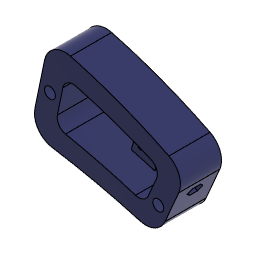
Tibia support middle v12 (Autodesk Fusion 360 design; units mm, degrees)
Autodesk Fusion 360 part; units mm, degrees
sketch "Sketch1" plane through (0, 0, 0) normal (0, 1, 0) x (1, 0, 0)
  line L0 (159.1401, 45.7067) -> (169.6952, 30.6325) construction
  line L1 (-17.5, 10) -> (-10.1, 10)
  line L2 (-18.6, 18.5) -> (-18.6, -18.5)
  line L3 (-17.5, 10) -> (-18.6, 10)
  circle A0 centre (0, 0) radius 2.5
  line L4 (74.5974, 20.8368) -> (81.7385, -13.7478)
  arc A1 (38.4, 18.5) -> (169.9824, 51.1436) centre (38.4, 300.018) ccw
  line L5 (169.9824, 51.1436) -> (178.5861, 38.8564)
  arc A2 (37.3, 10) -> (161.7212, 42.0206) centre (37.3, 267.7398) ccw
  line L6 (-10.1, -10) -> (29.9, -10)
  line L7 (-10.1, 10) -> (-10.1, -10)
  line L8 (29.9, 10) -> (-10.1, 10)
  line L9 (-17.5, -10) -> (-18.6, -10)
  line L10 (-17.5, -10) -> (-17.5, 10)
  line L11 (29.9, -10) -> (29.9, 10)
  line L12 (38.4, -18.5) -> (38.4, 18.5) construction
  line L13 (161.7212, 42.0206) -> (167.1141, 34.3187)
  line L14 (82.53, 21.9804) -> (89.5169, -11.8572)
  line L15 (9.9, -10) -> (9.9, -18.5) construction
  arc A3 (38.4, -18.5) -> (178.5861, 38.8564) centre (38.4, 181.4943) ccw
  line L16 (124.5058, 8.7395) -> (125.8994, 25.7068) construction
  line L17 (0, 0) -> (174.2843, 45) construction
  line L18 (-18.6, -18.5) -> (38.4, -18.5)
  line L19 (115.6359, 29.3023) -> (127.2705, 2.3303)
  line L20 (-10.1, -10) -> (-17.5, -10)
  line L21 (-10.1, 10) -> (-10.1, -10)
  line L22 (169.6952, 30.6325) -> (169.9824, 51.1436) construction
  line L23 (29.9, 10) -> (29.9, -10)
  line L24 (123.3477, 31.6223) -> (134.3836, 6.0382)
  arc A4 (37.3, -10) -> (167.1141, 34.3187) centre (37.3, 202.279) ccw
  line L25 (29.9, -10) -> (37.3, -10)
  line L26 (9.9, 10) -> (9.9, 18.5) construction
  line L27 (159.1401, 45.7067) -> (178.5861, 38.8564) construction
  line L28 (37.3, -10) -> (37.3, 10)
  line L29 (80.0659, -5.6475) -> (84.1183, 14.2879) construction
  line L30 (37.3, 10) -> (29.9, 10)
  line L31 (38.4, 18.5) -> (-18.6, 18.5)
  circle A5 centre (82.0921, 4.3202) radius 2.1
  circle A6 centre (125.2026, 17.2232) radius 2.1
  circle A7 centre (123.6183, 20.8961) radius 2.1
  point P0 (125.2026, 17.2232)
  point P1 (174.2843, 45)
  point P2 (37.3, 0)
  point P3 (82.0921, 4.3202)
  point P4 (-6.8918, -8.1801)
  point P5 (169.8534, 41.9327)
  point P6 (9.9, 13.85)
  dimension "d1" = 5
  dimension "d2" = 10.1
  dimension "d3" = 40
  dimension "d4" = 20
  dimension "d5" = 10
  dimension "d6" = 7.4
  dimension "d7" = 8.5
  dimension "d8" = 8.5
  dimension "d9" = 8.5
  dimension "d10" = 8.5
  dimension "d11" = 180
  dimension "d12" = 45
  dimension "d13" = 35
  dimension "d14" = 15
  dimension "d15" = 12
  dimension "d16" = 4.5
  dimension "d17" = 4.5
  dimension "d18" = 8
  dimension "d19" = 8
  dimension "d20" = 45
  dimension "d21" = 45
  dimension "d22" = 11.667
  dimension "d23" = 11.667
  dimension "d24" = 27.7
  dimension "d25" = 13.85
  dimension "d32" = 4.2
  dimension "d53" = 4
  dimension "d54" = 4
  constraint coincident A0.centre L17.start
  constraint horizontal L6
  constraint vertical L11
  constraint horizontal L8
  constraint vertical L21
  constraint horizontal L20
  constraint vertical L10
  constraint horizontal L1
  constraint vertical L7
  constraint horizontal L25
  constraint vertical L28
  constraint horizontal L30
  constraint vertical L23
  constraint coincident L1.end L7.start
  constraint coincident L8.start L11.end
  constraint equal L20 L25
  constraint horizontal L18
  constraint vertical L12
  constraint horizontal L31
  constraint vertical L2
  constraint coincident P1 L5
  constraint tangent A3 L18
  constraint tangent A1 L31
  constraint midpoint P1 L5
  constraint coincident P1 L17.end
  constraint parallel L0 L5
  constraint coincident L13.end L0
  constraint tangent A4 L25
  constraint coincident A2.end L0
  constraint tangent A2 L30
  constraint coincident L0.end A3
  constraint coincident L0.start A1
  constraint coincident L29.start A4
  constraint coincident L29.end A2
  constraint parallel L4 L14
  constraint coincident L16.start A4
  constraint coincident L16.end A2
  constraint parallel L19 L24
  constraint midpoint P3 L29
  constraint midpoint P0 L16
  constraint midpoint P2 L28
  constraint coincident L9.end L2
  constraint perpendicular L2 L9
  constraint coincident L3.end L2
  constraint perpendicular L2 L3
  constraint midpoint L15.start L6
  constraint midpoint L15.end L18
  constraint midpoint L26.start L8
  constraint midpoint L26.end L31
  constraint coincident P5 L27
  constraint coincident P5 L22
  constraint coincident P6 L26
  constraint coincident L29.start L4
  constraint coincident L29.end L14
  constraint coincident A3 L19.end
  constraint coincident L16.start L19
  constraint coincident A1 L19.start
  constraint coincident A1 L24.start
  constraint coincident L16.end L24
  constraint coincident A3 L4.end
  constraint coincident A3 L14.end
  constraint coincident A1 L4.start
  constraint coincident A1 L14.start
  constraint coincident A3 L24.end
  constraint coincident P3 A5.centre
  constraint coincident P0 A6.centre
  constraint equal A5 A6
  constraint equal A5 A7
  measures "d1" diameter of A0
  measures "d2" distance of A0.centre L21
  measures "d3" distance of L6.start L6.end
  measures "d4" distance of L8.start L6.end
  measures "d5" distance of A0.centre L6
  measures "d6" distance of L6.start L9.start
  measures "d7" distance of L2 L7
  measures "d8" distance of L11 L12
  measures "d9" distance of L8 L31
  measures "d10" distance of L6 L18
  measures "d11" distance of A0.centre P1
  measures "d12" vertical distance of P1 A0.centre
  measures "d13" angle of L2 L5
  measures "d14" distance of L5.end A1.end
  measures "d15" distance of L0 L5
  measures "d16" distance of L0.end L13.end
  measures "d17" distance of A2.end L0.start
  measures "d18" distance of L4 L14
  measures "d19" distance of L19 L24
  measures "d20" distance of P2 P3
  measures "d21" distance of P0 P3
  measures "d22" angle of L4 L28
  measures "d23" angle of L14 L19
  measures "d24" distance of P4 P6
  measures "d25" vertical distance of A0.centre P6
  measures "d32" diameter of A5
  measures "d53" distance of L24 A7.centre
  measures "d54" distance of P0 A7.centre
  measures "d57" angle of P2
extrude "Extrude1" add sketch "Sketch1" along normal blind 15.75 contours L4 A2 L14 A4 | L4 A1 A2 L14 | L4 L14 A3 A4 | A1 A2 L14 L19 | L14 A3 L19 A4 | A1 A2 L19 L24 | A2 L19 L24 A4 | A3 L19 L24 A4 | A6 A7 picked at (125.6121, 16.5727)
fillet "Fillet1" radius 4 4 edges at (84.1183, 7.875, -14.2879) (87.8714, 7.875, 3.8882) (124.5058, 7.875, -8.7395) (118.3255, 7.875, -23.0672)
fillet "Fillet2" radius 8 4 edges at (81.7385, 7.875, 13.7478) (74.5974, 7.875, -20.8368) (123.3477, 7.875, -31.6223) (134.3836, 7.875, -6.0382)
sketch "Sketch3" plane through (0, 15.75, 0) normal (0, 1, 0) x (-1, 0, 0)
  arc A0 (-127.668, -2.528) -> (-131.4429, -12.8555) centre (-124.0972, -9.6868) ccw
  line L0 (-131.4429, -12.8555) -> (-126.1762, -25.0651)
  arc A1 (-126.1762, -25.0651) -> (-116.608, -29.5815) centre (-118.8305, -21.8964) ccw
  arc A2 (-82.8853, -22.037) -> (-116.608, -29.5815) centre (-38.4, -300.018) ccw
  arc A3 (-82.8853, -22.037) -> (-76.3147, -12.5198) centre (-84.1494, -14.1375) ccw
  line L1 (-76.3147, -12.5198) -> (-80.0619, 5.6279)
  arc A4 (-80.0619, 5.6279) -> (-89.959, 11.7397) centre (-87.8966, 4.0101) ccw
  arc A5 (-89.959, 11.7397) -> (-127.668, -2.528) centre (-38.4, -181.4943) ccw
  circle A6 centre (-82.0921, -4.3202) radius 2.1
  arc A7 (-88.0674, -15.0493) -> (-114.8897, -21.9561) centre (-37.3, -267.7398) ccw
  arc A8 (-119.7668, -19.726) -> (-114.8897, -21.9561) centre (-116.0939, -18.1416) ccw
  line L2 (-119.7668, -19.726) -> (-122.9321, -12.3879)
  arc A9 (-120.8332, -7.1263) -> (-122.9321, -12.3879) centre (-119.2592, -10.8036) ccw
  arc A10 (-91.9713, 2.8391) -> (-120.8332, -7.1263) centre (-37.3, -202.279) ccw
  arc A11 (-87.0237, -0.2171) -> (-91.9713, 2.8391) centre (-90.9411, -1.026) ccw
  line L3 (-87.0237, -0.2171) -> (-84.9379, -10.3188)
  arc A12 (-88.0674, -15.0493) -> (-84.9379, -10.3188) centre (-88.8553, -11.1277) ccw
  line L4 (-114.8965, -4.6907) -> (-110.5283, -20.6216)
  line L5 (-110.5812, -20.4287) -> (-103.5285, -18.4949)
  line L6 (-103.5285, -18.4949) -> (-107.0323, -5.7165)
  line L7 (-107.0323, -5.7165) -> (-114.085, -7.6503)
  line L8 (-115.832, -5.0606) -> (-111.4868, -20.9076)
  line L9 (-107.071, -1.7936) -> (-102.5208, -18.3885)
  circle A13 centre (-107.8275, -9.4342) radius 1
  circle A14 centre (-106.1087, -15.7028) radius 1
  line L10 (-107.8275, -9.4342) -> (-106.1087, -15.7028)
  circle A15 centre (-123.6183, -20.8961) radius 2.1
  point P0 (-110.5283, -20.6216)
  point P1 (-106.9681, -12.5685)
  dimension "d33" = 8
  dimension "d34" = 0.2
  dimension "d35" = 10
  dimension "d36" = 13.25
  dimension "d37" = 7.313
  dimension "d38" = 1
  dimension "d39" = 1
  dimension "d40" = 6.5
  dimension "d41" = 6.625
  dimension "d42" = 1.75
  dimension "d43" = 2
  constraint coincident L4 L5.start
  constraint perpendicular L4 L5
  constraint coincident L4 L7.end
  constraint perpendicular L6 L7
  constraint perpendicular L4 L7
  constraint coincident L4 P0
  constraint coincident A7 P0
  constraint parallel L4 L8
  constraint parallel L6 L9
  constraint coincident A10 L8.start
  constraint coincident A10 L4.start
  constraint coincident A10 L9.start
  constraint coincident A7 L9.end
  constraint coincident A7 L8.end
  constraint coincident A13.centre L10.start
  constraint coincident A14.centre L10.end
  constraint parallel L6 L10
  constraint midpoint L10 P1
  constraint equal A13 A14
  measures "d33" angle of L2 L4
  measures "d34" distance of L5 P0
  measures "d35" distance of L2 L7.end
  measures "d36" distance of L5.end L6.end
  measures "d37" distance of L6.end L7.end
  measures "d38" distance of L4 L8
  measures "d39" distance of L6 L9
  measures "d40" distance of A13.centre A14.centre
  measures "d41" distance of L7 P1
  measures "d42" distance of L6 L10
  measures "d43" diameter of A13
extrude "Extrude2" add sketch "Sketch3" against normal blind 5 contours A7 A10 L4 L5 L6 L7 L9 | A7 A10 L4 L8 | L4 L5 L6 L7
ref_plane "WorkPlane1" through (126.1762, 7.875, -25.0651) normal (-0.819152, 0, 0.573576) x (0, -1, 0)
sketch "Sketch5" plane through (96.4423, 0, -67.5296) normal (-0.819152, 0, 0.573576) x (0, -1, 0)
  line L0 (-6.375, 62.3396) -> (-9.375, 62.3396)
  line L1 (-9.375, 62.3396) -> (-9.375, 59.3396)
  line L2 (-9.375, 59.3396) -> (-6.375, 59.3396)
  line L3 (-6.375, 59.3396) -> (-6.375, 62.3396)
  line L4 (-9.375, 62.3396) -> (-10.875, 60.8396)
  line L5 (-10.875, 60.8396) -> (-9.375, 59.3396)
  line L6 (-6.375, 62.3396) -> (-4.875, 60.8396)
  line L7 (-4.875, 60.8396) -> (-6.375, 59.3396)
  line L8 (-7.875, 63.0141) -> (-7.875, 45.7648) construction
  line L9 (0, 51.8396) -> (0, 64.862)
  line L10 (-15.75, 51.8396) -> (0, 51.8396)
  dimension "d57" = 45
  dimension "d58" = 45
  dimension "d59" = 3
  dimension "d60" = 7.875
  dimension "d61" = 1.5
  dimension "d62" = 7.5
  constraint horizontal L0
  constraint vertical L1
  constraint horizontal L2
  constraint vertical L3
  constraint parallel L5 L6
  constraint parallel L4 L7
  constraint equal L0 L1
  constraint vertical L8
  measures "d57" angle of L1 L4
  measures "d58" angle of L3 L6
  measures "d59" distance of L0.start L0.end
  measures "d60" distance of L8 L9
  measures "d61" distance of L1 L8
  measures "d62" distance of L2 L10
extrude "Extrude4" cut sketch "Sketch5" along normal blind 17
equation "d41 = d36 / 2"
equation "d53 = d19 / 2"
equation "d56 = 90 deg - 35 deg"
equation "d60 = ( 15.75 / 2 ) * 1 mm"
equation "d61 = d59 / 2"
